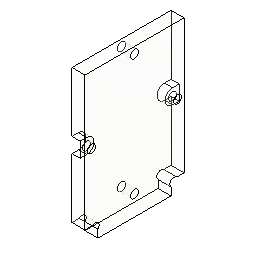
RampBack v5 (Autodesk Fusion 360 design; units mm, degrees)
Autodesk Fusion 360 part; units mm, degrees
sketch "Sketch1" plane through (0, 0, 0) normal (1, 0, 0) x (0, 1, 0)
  line L0 (-18.3, 27.3) -> (18.3, 27.3)
  line L1 (18.3, 27.3) -> (18.3, -22.3)
  line L2 (13.5, -27.3) -> (-13.5, -27.3)
  line L3 (-18.3, -22.3) -> (-18.3, 27.3)
  line L4 (0, 0) -> (0, 27.3) construction
  line L5 (-13.5, 27.3) -> (-13.5, -22.3) construction
  line L6 (13.5, 27.3) -> (13.5, -22.3) construction
  line L7 (-18.3, 22.5) -> (18.3, 22.5) construction
  line L8 (-18.3, -17.5) -> (18.3, -17.5) construction
  line L9 (-13.5, -22.3) -> (13.5, -22.3) construction
  line L10 (-18.3, 2.5) -> (18.3, 2.5) construction
  line L11 (0, 0) -> (0, -19.9) construction
  circle A0 centre (0, -19.9) radius 1.5
  circle A1 centre (-15.9, 2.5) radius 1.5
  circle A2 centre (15.9, 2.5) radius 1.5
  circle A3 centre (0, 24.9) radius 1.5
  line L12 (-18.3, -22.3) -> (-15.6213, -22.3)
  line L13 (-13.5, -24.4213) -> (-13.5, -27.3)
  line L14 (13.5, -24.4213) -> (13.5, -27.3)
  line L15 (15.6213, -22.3) -> (18.3, -22.3)
  line L16 (-18.3, -27.3) -> (-18.3, -22.3) construction
  line L17 (-13.5, -27.3) -> (-18.3, -27.3) construction
  line L18 (18.3, -27.3) -> (13.5, -27.3) construction
  line L19 (0, 0) -> (18.3, 0)
  line L20 (18.3, -22.3) -> (18.3, -27.3) construction
  line L21 (-13.5, -22.3) -> (-14.5607, -23.3607) construction
  arc A4 (-13.5, -24.4213) -> (-15.6213, -22.3) centre (-14.5607, -23.3607) ccw
  arc A5 (-15.6213, -22.3) -> (-13.5, -24.4213) centre (-14.5607, -23.3607) ccw construction
  line L22 (-13.5, -22.3) -> (-13.5, -24.4213) construction
  line L23 (-15.6213, -22.3) -> (-13.5, -22.3) construction
  line L24 (13.5, -22.3) -> (14.5607, -23.3607) construction
  arc A6 (15.6213, -22.3) -> (13.5, -24.4213) centre (14.5607, -23.3607) ccw
  arc A7 (13.5, -24.4213) -> (15.6213, -22.3) centre (14.5607, -23.3607) ccw construction
  line L25 (13.5, -22.3) -> (15.6213, -22.3) construction
  line L26 (13.5, -22.3) -> (13.5, -24.4213) construction
  line L27 (-15.9, -0.25) -> (-18.3, -0.25)
  line L28 (-15.9, 5.25) -> (-18.3, 5.25)
  arc A8 (-15.9, -0.25) -> (-15.9, 5.25) centre (-15.9, 2.5) ccw
  arc A9 (-15.9, 5.25) -> (-18.3, 3.8426) centre (-15.9, 2.5) ccw construction
  arc A10 (-18.3, 3.8426) -> (-18.3, 1.1574) centre (-15.9, 2.5) ccw construction
  arc A11 (-18.3, 1.1574) -> (-15.9, -0.25) centre (-15.9, 2.5) ccw construction
  line L29 (15.9, 5.25) -> (18.3, 5.25)
  line L30 (15.9, -0.25) -> (18.3, -0.25)
  arc A12 (15.9, -0.25) -> (15.9, 5.25) centre (15.9, 2.5) ccw construction
  arc A13 (14.7544, 0) -> (15.9, -0.25) centre (15.9, 2.5) ccw
  arc A14 (13.5, 1.1574) -> (14.7544, 0) centre (15.9, 2.5) ccw
  arc A15 (13.15, 2.5) -> (13.5, 1.1574) centre (15.9, 2.5) ccw
  arc A16 (13.5, 3.8426) -> (13.15, 2.5) centre (15.9, 2.5) ccw
  arc A17 (15.9, 5.25) -> (13.5, 3.8426) centre (15.9, 2.5) ccw
  point P0 (18.3, 0)
  dimension "d20" = 4.8
  dimension "d21" = 4.8
  dimension "d22" = 4.8
  dimension "d23" = 27
  dimension "d24" = 4.8
  dimension "d25" = 5
  dimension "d26" = 40
  dimension "d27" = 20
  dimension "d28" = 2.4
  dimension "d29" = 3
  dimension "d30" = 3
  dimension "d31" = 3
  dimension "d32" = 3
  dimension "d33" = 2.4
  dimension "d34" = 2.4
  dimension "d35" = 2.4
  dimension "d38" = 2.5
  dimension "d39" = 1.5
  dimension "d40" = 45
  dimension "d41" = 3
  dimension "d42" = 1.5
  dimension "d43" = 45
  dimension "d44" = 3
  dimension "d45" = 5.5
  dimension "d46" = 5.5
  constraint horizontal L0
  constraint vertical L1
  constraint horizontal L2
  constraint vertical L3
  constraint coincident L4.start L11.start
  constraint midpoint L0 L4.end
  constraint vertical L4
  constraint coincident L0 L5.start
  constraint perpendicular L2 L5
  constraint coincident L0 L6.start
  constraint perpendicular L2 L6
  constraint coincident L3 L7.start
  constraint coincident L1 L7.end
  constraint perpendicular L1 L7
  constraint coincident L3 L8.start
  constraint coincident L1 L8.end
  constraint perpendicular L1 L8
  constraint perpendicular L1 L9
  constraint coincident L3 L10.start
  constraint coincident L1 L10.end
  constraint perpendicular L1 L10
  constraint perpendicular L8 L11
  constraint coincident L11.end A0.centre
  constraint coincident L10 A1.centre
  constraint coincident L10 A2.centre
  constraint coincident L4 A3.centre
  constraint perpendicular L1 L12
  constraint perpendicular L2 L13
  constraint perpendicular L2 L14
  constraint perpendicular L1 L15
  constraint vertical L16
  constraint horizontal L17
  constraint horizontal L18
  constraint coincident L1 P0
  constraint coincident P0 L19.end
  constraint perpendicular L1 L19
  constraint vertical L20
  constraint coincident L21.end A4.centre
  constraint concentric A4 A5
  constraint perpendicular L2 L22
  constraint perpendicular L1 L23
  constraint coincident L24.end A6.centre
  constraint concentric A6 A7
  constraint perpendicular L1 L25
  constraint perpendicular L2 L26
  constraint concentric A1 A8
  constraint coincident L3 L27.end
  constraint tangent L27 A8
  constraint horizontal L27
  constraint coincident L3 L28.end
  constraint perpendicular L3 L28
  constraint tangent L28 A8
  constraint coincident L3 A9.end
  constraint concentric A8 A9
  constraint coincident L3 A10.end
  constraint concentric A8 A10
  constraint concentric A8 A11
  constraint concentric A2 A12
  constraint coincident L1 L29.end
  constraint perpendicular L1 L29
  constraint tangent L29 A12
  constraint coincident L1 L30.end
  constraint horizontal L30
  constraint tangent L30 A12
  constraint coincident L19 A13.start
  constraint concentric A12 A13
  constraint coincident L6 A14.start
  constraint concentric A12 A14
  constraint coincident L10 A15.start
  constraint concentric A12 A15
  constraint coincident L6 A16.start
  constraint concentric A12 A16
  constraint concentric A12 A17
  measures "d20" distance of L3 L5
  measures "d21" distance of L1 L6
  measures "d22" distance of L0 L7
  measures "d23" distance of L5 L6
  measures "d24" distance of L8 L9
  measures "d25" distance of L2 L9
  measures "d26" distance of L7 L8
  measures "d27" distance of L7 L10
  measures "d28" distance of L8 L11.end
  measures "d29" diameter of A0
  measures "d30" diameter of A1
  measures "d31" diameter of A2
  measures "d32" diameter of A3
  measures "d33" distance of L0 A3.centre
  measures "d34" distance of L3 A1.centre
  measures "d35" distance of L1 A2.centre
  measures "d38" distance of L10 P0
  measures "d39" distance of L5.end L21.end
  measures "d40" angle of L12 L21
  measures "d41" diameter of A4
  measures "d42" distance of L6.end L24.end
  measures "d43" angle of L15 L24
  measures "d44" diameter of A6
  measures "d45" diameter of A8
  measures "d46" diameter of A12
extrude "Extrude1" add sketch "Sketch1" along normal blind 4.8
extrude "Extrude2" cut sketch "Sketch1" along normal blind 3 contours L3 L27 L28 A8 | L1 L19 L29 A14 A15 A16 A17 | L1 L19 L30 A13
